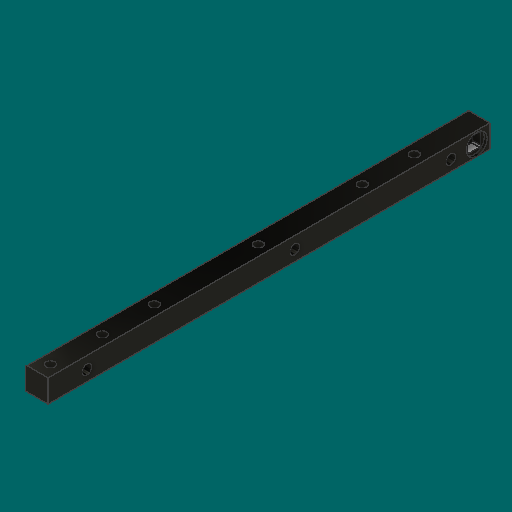
# Autodesk Inventor part: Intake_BOX
Saved by Autodesk Inventor 2025.2 (Build 292293000, 293)
## iProperties
Created: 2025-01-16
Part Number: Intake_BOX
Material: Generic
Document SubType Name: Modeling
Designer: Collin
Density: 1 g/cm^3
Appearance: Default
Author: Collin
Autodesk Inventor part; units mm, degrees
ref_plane "YZ Plane" through (0, 0, 0) normal (1, 0, 0) x (0, 1, 0)
ref_plane "XZ Plane" through (0, 0, 0) normal (0, 1, 0) x (-1, 0, 0)
ref_plane "XY Plane" through (0, 0, 0) normal (0, 0, 1) x (1, 0, 0)
sketch "Sketch1" plane through (0, 0, 0) normal (0, 1, 0) x (-1, 0, 0)
  point P0 (0, 0)
sketch "Sketch2" plane through (0, 0, 0) normal (0, 0, 1) x (1, 0, 0)
  line L0 (-7.0379, 7.3301) -> (-7.0379, 5.7426)
  line L1 (-7.0379, 7.3301) -> (-16.3407, 7.3301)
  line L2 (-16.3407, 7.3301) -> (-16.3407, 5.7426)
  line L3 (-16.3407, 5.7426) -> (-7.0379, 5.7426)
  arc A0 (-16.3407, 7.3301) -> (-18.7219, 4.9488) centre (-16.3407, 4.9488) ccw
  line L4 (-17.1344, 4.9488) -> (-18.7219, 4.9488)
  arc A1 (-16.3407, 5.7426) -> (-17.1344, 4.9488) centre (-16.3407, 4.9488) ccw
  line L5 (-16.3407, 7.3301) -> (-16.3407, 5.7426)
  arc A2 (-16.3407, 7.3301) -> (-18.7219, 4.9488) centre (-16.3407, 4.9488) ccw
  line L6 (-17.1344, 4.9488) -> (-18.7219, 4.9488)
  arc A3 (-16.3407, 5.7426) -> (-17.1344, 4.9488) centre (-16.3407, 4.9488) ccw
  line L7 (-7.0379, 7.3301) -> (-7.0379, 5.7426)
  line L8 (-7.0379, 7.3301) -> (-16.3407, 7.3301)
  line L9 (-16.3407, 5.7426) -> (-7.0379, 5.7426)
  line L10 (-18.7219, 2.1231) -> (-17.1344, 2.1231)
  line L11 (-17.1344, -4.3539) -> (-18.7219, -4.3539)
  line L12 (-17.1344, -4.3539) -> (-17.1344, 4.9488)
  line L13 (-17.1344, 4.9488) -> (-18.7219, 4.9488)
  line L14 (-18.7219, -4.3539) -> (-18.7219, 4.9488)
  line L15 (-17.1344, -5.3699) -> (-17.1344, -4.3539)
  line L16 (-17.1344, -4.3539) -> (-18.7219, -4.3539)
  line L17 (-18.7219, -4.3539) -> (-18.7219, -5.3699)
  line L18 (-18.7219, -5.3699) -> (-17.1344, -5.3699)
  line L19 (-6.0219, 7.3301) -> (-7.0379, 7.3301)
  line L20 (-7.0379, 7.3301) -> (-7.0379, 5.7426)
  line L21 (-7.0379, 5.7426) -> (-6.0219, 5.7426)
  line L22 (-6.0219, 5.7426) -> (-6.0219, 7.3301)
  line L23 (-17.1344, -5.3699) -> (-6.0219, -5.3699)
  line L24 (-6.0219, -5.3699) -> (-6.0219, 5.7426)
  point P0 (0, 0)
  point P1 (-18.7219, 0.9801)
  constraints: 50 end point, 8 point on circle, 4 centre point, 1 perpendicular
extrude "Extrusion1" add sketch "Sketch2" against normal blind 215.9 contours L21 L24 L23 L15 L12 A1 L3
sketch "Sketch3" plane through (-16.3407, 5.7426, 0) normal (0, 1, 0) x (1, 0, 0)
  line L0 (2.8257, 196.6074) -> (2.8257, 197.0926)
  line L1 (7.4485, 197.0926) -> (7.4485, 196.6074)
  line L2 (5.3798, 194.5386) -> (4.8945, 194.5386)
  line L3 (0, 215.9) -> (9.3027, 215.9)
  line L4 (0, 215.9) -> (0, 191.6657)
  line L5 (0, 191.6657) -> (1.1657, 190.5)
  line L6 (1.1657, 190.5) -> (0, 189.3343)
  line L7 (0, 189.3343) -> (0, 128.1657)
  line L8 (0, 128.1657) -> (1.1657, 127)
  line L9 (1.1657, 127) -> (0, 125.8343)
  line L10 (0, 125.8343) -> (0, 64.6657)
  line L11 (0, 64.6657) -> (1.1657, 63.5)
  line L12 (1.1657, 63.5) -> (0, 62.3343)
  line L13 (9.3027, 0) -> (0, 0)
  line L14 (10.3187, 61.468) -> (10.3187, 1.016)
  line L15 (10.3187, 61.468) -> (8.2867, 63.5)
  line L16 (8.2867, 63.5) -> (10.3187, 65.532)
  line L17 (10.3187, 124.968) -> (10.3187, 65.532)
  line L18 (10.3187, 124.968) -> (8.2867, 127)
  line L19 (8.2867, 127) -> (10.3187, 129.032)
  line L20 (10.3187, 188.468) -> (10.3187, 129.032)
  line L21 (10.3187, 188.468) -> (8.2867, 190.5)
  line L22 (8.2867, 190.5) -> (10.3187, 192.532)
  line L23 (10.3187, 214.884) -> (10.3187, 192.532)
  line L24 (-0.7938, 0) -> (0, 0)
  line L25 (0, 215.9) -> (10.3187, 215.9) projected
  line L26 (0, 215.9) -> (-0.7938, 215.9) projected
  line L27 (0, 0) -> (-0.7938, 0) projected
  line L28 (0, 0) -> (0, 215.9) projected
  line L29 (-0.7938, 215.9) -> (0, 215.9) projected
  line L30 (-0.7938, 0) -> (-0.7938, 215.9) projected
  line L31 (10.3187, 0) -> (0, 0) projected
  line L32 (10.3187, 0) -> (10.3187, 215.9) projected
  line L33 (0, 215.9) -> (10.3187, 215.9) projected
  line L34 (0, 0) -> (0, 215.9) projected
  line L35 (9.3027, 215.9) -> (10.3187, 215.9)
  line L36 (10.3187, 215.9) -> (10.3187, 214.884)
  line L37 (0, 62.3343) -> (0, 21.3614)
  line L38 (0, 16.7386) -> (0, 0)
  circle A0 centre (5.1371, 209.55) radius 2.161
  circle A1 centre (5.1371, 196.85) radius 2.161
  circle A2 centre (5.1371, 184.15) radius 2.161
  circle A3 centre (5.1371, 171.45) radius 2.161
  circle A4 centre (5.1371, 158.75) radius 2.161
  circle A5 centre (5.1371, 146.05) radius 2.161
  circle A6 centre (5.1371, 133.35) radius 2.161
  circle A7 centre (5.1371, 120.65) radius 2.161
  circle A8 centre (5.1371, 107.95) radius 2.161
  circle A9 centre (5.1371, 95.25) radius 2.161
  circle A10 centre (5.1371, 82.55) radius 2.161
  circle A11 centre (5.1371, 69.85) radius 2.161
  circle A12 centre (5.1371, 57.15) radius 2.161
  circle A13 centre (5.1371, 44.45) radius 2.161
  circle A14 centre (5.1371, 31.75) radius 2.161
  circle A15 centre (5.1371, 19.05) radius 2.161
  circle A16 centre (5.1371, 6.35) radius 2.161
  point P0 (16.3407, 0)
  dimension "d9" = 12.7
  constraints: 58 end point, 17 centre point, 1 horizontal, 1 perpendicular, 1 point on line, 1 vertical, 32 other
  measures "d9" distance of A0.centre A1.centre
extrude "Extrusion2" cut sketch "Sketch3" along normal mid plane 215.9 contours A2 | A4 | A8 | A12 | A14 | A16
sketch "Sketch4" plane through (-6.0219, -5.3699, 0) normal (1, 0, 0) x (0, 0, -1)
  line L0 (0, 0) -> (0, 11.1125)
  line L1 (0, 0) -> (215.9, 0)
  line L2 (215.9, 11.1125) -> (215.9, 0)
  line L3 (0, 11.1125) -> (215.9, 11.1125)
  arc A0 (4.5466, 7.493) -> (4.0386, 6.985) centre (4.5466, 6.985) ccw
  line L4 (4.5466, 7.493) -> (8.1534, 7.493)
  arc A1 (8.6614, 6.985) -> (8.1534, 7.493) centre (8.1534, 6.985) ccw
  line L5 (8.6614, 6.985) -> (8.6614, 3.3782)
  arc A2 (8.1534, 2.8702) -> (8.6614, 3.3782) centre (8.1534, 3.3782) ccw
  line L6 (8.1534, 2.8702) -> (4.5466, 2.8702)
  arc A3 (4.0386, 3.3782) -> (4.5466, 2.8702) centre (4.5466, 3.3782) ccw
  line L7 (4.0386, 3.3782) -> (4.0386, 6.985)
  arc A4 (29.9466, 7.493) -> (29.4386, 6.985) centre (29.9466, 6.985) ccw
  line L8 (29.9466, 7.493) -> (33.5534, 7.493)
  arc A5 (34.0614, 6.985) -> (33.5534, 7.493) centre (33.5534, 6.985) ccw
  line L9 (34.0614, 6.985) -> (34.0614, 3.3782)
  arc A6 (33.5534, 2.8702) -> (34.0614, 3.3782) centre (33.5534, 3.3782) ccw
  line L10 (33.5534, 2.8702) -> (29.9466, 2.8702)
  arc A7 (29.4386, 3.3782) -> (29.9466, 2.8702) centre (29.9466, 3.3782) ccw
  line L11 (29.4386, 3.3782) -> (29.4386, 6.985)
  arc A8 (42.6466, 7.493) -> (42.1386, 6.985) centre (42.6466, 6.985) ccw
  line L12 (42.6466, 7.493) -> (46.2534, 7.493)
  arc A9 (46.7614, 6.985) -> (46.2534, 7.493) centre (46.2534, 6.985) ccw
  line L13 (46.7614, 6.985) -> (46.7614, 3.3782)
  arc A10 (46.2534, 2.8702) -> (46.7614, 3.3782) centre (46.2534, 3.3782) ccw
  line L14 (46.2534, 2.8702) -> (42.6466, 2.8702)
  arc A11 (42.1386, 3.3782) -> (42.6466, 2.8702) centre (42.6466, 3.3782) ccw
  line L15 (42.1386, 3.3782) -> (42.1386, 6.985)
  arc A12 (55.3466, 7.493) -> (54.8386, 6.985) centre (55.3466, 6.985) ccw
  line L16 (55.3466, 7.493) -> (58.9534, 7.493)
  arc A13 (59.4614, 6.985) -> (58.9534, 7.493) centre (58.9534, 6.985) ccw
  line L17 (59.4614, 6.985) -> (59.4614, 3.3782)
  arc A14 (58.9534, 2.8702) -> (59.4614, 3.3782) centre (58.9534, 3.3782) ccw
  line L18 (58.9534, 2.8702) -> (55.3466, 2.8702)
  arc A15 (54.8386, 3.3782) -> (55.3466, 2.8702) centre (55.3466, 3.3782) ccw
  line L19 (54.8386, 3.3782) -> (54.8386, 6.985)
  arc A16 (68.0466, 7.493) -> (67.5386, 6.985) centre (68.0466, 6.985) ccw
  line L20 (68.0466, 7.493) -> (71.6534, 7.493)
  arc A17 (72.1614, 6.985) -> (71.6534, 7.493) centre (71.6534, 6.985) ccw
  line L21 (72.1614, 6.985) -> (72.1614, 3.3782)
  arc A18 (71.6534, 2.8702) -> (72.1614, 3.3782) centre (71.6534, 3.3782) ccw
  line L22 (71.6534, 2.8702) -> (68.0466, 2.8702)
  arc A19 (67.5386, 3.3782) -> (68.0466, 2.8702) centre (68.0466, 3.3782) ccw
  line L23 (67.5386, 3.3782) -> (67.5386, 6.985)
  arc A20 (80.7466, 7.493) -> (80.2386, 6.985) centre (80.7466, 6.985) ccw
  line L24 (80.7466, 7.493) -> (84.3534, 7.493)
  arc A21 (84.8614, 6.985) -> (84.3534, 7.493) centre (84.3534, 6.985) ccw
  line L25 (84.8614, 6.985) -> (84.8614, 3.3782)
  arc A22 (84.3534, 2.8702) -> (84.8614, 3.3782) centre (84.3534, 3.3782) ccw
  line L26 (84.3534, 2.8702) -> (80.7466, 2.8702)
  arc A23 (80.2386, 3.3782) -> (80.7466, 2.8702) centre (80.7466, 3.3782) ccw
  line L27 (80.2386, 3.3782) -> (80.2386, 6.985)
  arc A24 (93.4466, 7.493) -> (92.9386, 6.985) centre (93.4466, 6.985) ccw
  line L28 (93.4466, 7.493) -> (97.0534, 7.493)
  arc A25 (97.5614, 6.985) -> (97.0534, 7.493) centre (97.0534, 6.985) ccw
  line L29 (97.5614, 6.985) -> (97.5614, 3.3782)
  arc A26 (97.0534, 2.8702) -> (97.5614, 3.3782) centre (97.0534, 3.3782) ccw
  line L30 (97.0534, 2.8702) -> (93.4466, 2.8702)
  arc A27 (92.9386, 3.3782) -> (93.4466, 2.8702) centre (93.4466, 3.3782) ccw
  line L31 (92.9386, 3.3782) -> (92.9386, 6.985)
  arc A28 (106.1466, 7.493) -> (105.6386, 6.985) centre (106.1466, 6.985) ccw
  line L32 (106.1466, 7.493) -> (109.7534, 7.493)
  arc A29 (110.2614, 6.985) -> (109.7534, 7.493) centre (109.7534, 6.985) ccw
  line L33 (110.2614, 6.985) -> (110.2614, 3.3782)
  arc A30 (109.7534, 2.8702) -> (110.2614, 3.3782) centre (109.7534, 3.3782) ccw
  line L34 (109.7534, 2.8702) -> (106.1466, 2.8702)
  arc A31 (105.6386, 3.3782) -> (106.1466, 2.8702) centre (106.1466, 3.3782) ccw
  line L35 (105.6386, 3.3782) -> (105.6386, 6.985)
  line L36 (120.4074, 7.493) -> (120.8926, 7.493)
  arc A32 (131.5466, 7.493) -> (131.0386, 6.985) centre (131.5466, 6.985) ccw
  line L37 (131.5466, 7.493) -> (135.1534, 7.493)
  arc A33 (135.6614, 6.985) -> (135.1534, 7.493) centre (135.1534, 6.985) ccw
  line L38 (135.6614, 6.985) -> (135.6614, 3.3782)
  arc A34 (135.1534, 2.8702) -> (135.6614, 3.3782) centre (135.1534, 3.3782) ccw
  line L39 (135.1534, 2.8702) -> (131.5466, 2.8702)
  arc A35 (131.0386, 3.3782) -> (131.5466, 2.8702) centre (131.5466, 3.3782) ccw
  line L40 (131.0386, 3.3782) -> (131.0386, 6.985)
  arc A36 (144.2466, 7.493) -> (143.7386, 6.985) centre (144.2466, 6.985) ccw
  line L41 (144.2466, 7.493) -> (147.8534, 7.493)
  arc A37 (148.3614, 6.985) -> (147.8534, 7.493) centre (147.8534, 6.985) ccw
  line L42 (148.3614, 6.985) -> (148.3614, 3.3782)
  arc A38 (147.8534, 2.8702) -> (148.3614, 3.3782) centre (147.8534, 3.3782) ccw
  line L43 (147.8534, 2.8702) -> (144.2466, 2.8702)
  arc A39 (143.7386, 3.3782) -> (144.2466, 2.8702) centre (144.2466, 3.3782) ccw
  line L44 (143.7386, 3.3782) -> (143.7386, 6.985)
  arc A40 (156.9466, 7.493) -> (156.4386, 6.985) centre (156.9466, 6.985) ccw
  line L45 (156.9466, 7.493) -> (160.5534, 7.493)
  arc A41 (161.0614, 6.985) -> (160.5534, 7.493) centre (160.5534, 6.985) ccw
  line L46 (161.0614, 6.985) -> (161.0614, 3.3782)
  arc A42 (160.5534, 2.8702) -> (161.0614, 3.3782) centre (160.5534, 3.3782) ccw
  line L47 (160.5534, 2.8702) -> (156.9466, 2.8702)
  arc A43 (156.4386, 3.3782) -> (156.9466, 2.8702) centre (156.9466, 3.3782) ccw
  line L48 (156.4386, 3.3782) -> (156.4386, 6.985)
  arc A44 (169.6466, 7.493) -> (169.1386, 6.985) centre (169.6466, 6.985) ccw
  line L49 (169.6466, 7.493) -> (173.2534, 7.493)
  arc A45 (173.7614, 6.985) -> (173.2534, 7.493) centre (173.2534, 6.985) ccw
  line L50 (173.7614, 6.985) -> (173.7614, 3.3782)
  arc A46 (173.2534, 2.8702) -> (173.7614, 3.3782) centre (173.2534, 3.3782) ccw
  line L51 (173.2534, 2.8702) -> (169.6466, 2.8702)
  arc A47 (169.1386, 3.3782) -> (169.6466, 2.8702) centre (169.6466, 3.3782) ccw
  line L52 (169.1386, 3.3782) -> (169.1386, 6.985)
  arc A48 (182.3466, 7.493) -> (181.8386, 6.985) centre (182.3466, 6.985) ccw
  line L53 (182.3466, 7.493) -> (185.9534, 7.493)
  arc A49 (186.4614, 6.985) -> (185.9534, 7.493) centre (185.9534, 6.985) ccw
  line L54 (186.4614, 6.985) -> (186.4614, 3.3782)
  arc A50 (185.9534, 2.8702) -> (186.4614, 3.3782) centre (185.9534, 3.3782) ccw
  line L55 (185.9534, 2.8702) -> (182.3466, 2.8702)
  arc A51 (181.8386, 3.3782) -> (182.3466, 2.8702) centre (182.3466, 3.3782) ccw
  line L56 (181.8386, 3.3782) -> (181.8386, 6.985)
  arc A52 (207.7466, 7.493) -> (207.2386, 6.985) centre (207.7466, 6.985) ccw
  line L57 (207.7466, 7.493) -> (211.3534, 7.493)
  arc A53 (211.8614, 6.985) -> (211.3534, 7.493) centre (211.3534, 6.985) ccw
  line L58 (211.8614, 6.985) -> (211.8614, 3.3782)
  arc A54 (211.3534, 2.8702) -> (211.8614, 3.3782) centre (211.3534, 3.3782) ccw
  line L59 (211.3534, 2.8702) -> (207.7466, 2.8702)
  arc A55 (207.2386, 3.3782) -> (207.7466, 2.8702) centre (207.7466, 3.3782) ccw
  line L60 (207.2386, 3.3782) -> (207.2386, 6.985)
  line L61 (215.9, 10.3187) -> (215.9, 1.016)
  line L62 (215.9, 10.3187) -> (191.6657, 10.3187)
  line L63 (189.3343, 10.3187) -> (128.1657, 10.3187)
  line L64 (125.8343, 10.3187) -> (64.6657, 10.3187)
  line L65 (62.3343, 10.3187) -> (0, 10.3187)
  line L66 (0, 1.016) -> (0, 10.3187)
  line L67 (61.468, 0) -> (1.016, 0)
  line L68 (124.968, 0) -> (65.532, 0)
  line L69 (188.468, 0) -> (129.032, 0)
  line L70 (214.884, 0) -> (192.532, 0)
  line L71 (1.016, 12.7) -> (0, 12.7)
  line L72 (0, 12.7) -> (0, 11.1125)
  line L73 (0, 11.1125) -> (1.016, 11.1125)
  line L74 (1.016, 11.1125) -> (1.016, 12.7)
  spline S0 degree 3 poles (61.2372, 10.9075) (61.6029, 11.0379) (61.9686, 11.1125) (62.3343, 11.1125) knots -1 -1 -1 -1 0 0 0 0
  line L75 (0, 11.1125) -> (62.3343, 11.1125)
  line L76 (0, 10.3187) -> (0, 11.1125)
  line L77 (62.3343, 10.3187) -> (0, 10.3187)
  spline S1 degree 3 poles (62.3343, 10.3187) (61.9686, 10.5133) (61.6029, 10.7069) (61.2372, 10.8512) knots 0 0 0 0 1 1 1 1
  spline S2 degree 3 poles (61.2372, 10.8512) (61.2621, 10.861) (61.2871, 10.8706) (61.312, 10.88) knots 0 0 0 0 1 1 1 1
  spline S3 degree 3 poles (61.312, 10.88) (61.2871, 10.8894) (61.2621, 10.8985) (61.2372, 10.9075) knots 0 0 0 0 1 1 1 1
  line L78 (1.016, 11.1125) -> (1.016, 12.7)
  line L79 (61.468, 11.1125) -> (1.016, 11.1125)
  line L80 (61.468, 11.1125) -> (61.468, 12.7)
  line L81 (61.468, 12.7) -> (1.016, 12.7)
  line L82 (63.5, 11.1125) -> (61.468, 11.1125)
  line L83 (63.5, 12.7) -> (63.5, 11.1125)
  line L84 (61.468, 12.7) -> (63.5, 12.7)
  line L85 (61.468, 11.1125) -> (61.468, 12.7)
  line L86 (65.532, 11.1125) -> (63.5, 11.1125)
  line L87 (65.532, 12.7) -> (65.532, 11.1125)
  line L88 (63.5, 12.7) -> (65.532, 12.7)
  line L89 (63.5, 12.7) -> (63.5, 11.1125)
  line L90 (68.0466, 12.7) -> (68.0466, 11.1125)
  line L91 (124.968, 11.1125) -> (124.968, 12.7)
  line L92 (124.968, 12.7) -> (65.532, 12.7)
  line L93 (65.532, 12.7) -> (65.532, 11.1125)
  line L94 (124.968, 11.1125) -> (65.532, 11.1125)
  spline S4 degree 3 poles (124.7372, 10.9075) (125.1029, 11.0379) (125.4686, 11.1125) (125.8343, 11.1125) knots -1 -1 -1 -1 0 0 0 0
  line L95 (64.6657, 11.1125) -> (125.8343, 11.1125)
  spline S5 degree 3 poles (64.6657, 11.1125) (65.0314, 11.1125) (65.3971, 11.0379) (65.7628, 10.9075) knots -1 -1 -1 -1 0 0 0 0
  spline S6 degree 3 poles (65.7628, 10.9075) (65.7379, 10.8985) (65.7129, 10.8894) (65.688, 10.88) knots 0 0 0 0 1 1 1 1
  spline S7 degree 3 poles (65.688, 10.88) (65.7129, 10.8706) (65.7379, 10.861) (65.7628, 10.8512) knots 0 0 0 0 1 1 1 1
  spline S8 degree 3 poles (65.7628, 10.8512) (65.3971, 10.7069) (65.0314, 10.5133) (64.6657, 10.3187) knots 0 0 0 0 1 1 1 1
  line L96 (125.8343, 10.3187) -> (64.6657, 10.3187)
  spline S9 degree 3 poles (125.8343, 10.3187) (125.4686, 10.5133) (125.1029, 10.7069) (124.7372, 10.8512) knots 0 0 0 0 1 1 1 1
  spline S10 degree 3 poles (124.7372, 10.8512) (124.7621, 10.861) (124.7871, 10.8706) (124.812, 10.88) knots 0 0 0 0 1 1 1 1
  spline S11 degree 3 poles (124.812, 10.88) (124.7871, 10.8894) (124.7621, 10.8985) (124.7372, 10.9075) knots 0 0 0 0 1 1 1 1
  line L97 (129.032, 11.1125) -> (127, 11.1125)
  line L98 (129.032, 12.7) -> (129.032, 11.1125)
  line L99 (127, 12.7) -> (129.032, 12.7)
  line L100 (127, 12.7) -> (127, 11.1125)
  line L101 (127, 11.1125) -> (124.968, 11.1125)
  line L102 (127, 12.7) -> (127, 11.1125)
  line L103 (124.968, 12.7) -> (127, 12.7)
  line L104 (124.968, 11.1125) -> (124.968, 12.7)
  line L105 (129.032, 12.7) -> (129.032, 11.1125)
  line L106 (188.468, 11.1125) -> (129.032, 11.1125)
  line L107 (188.468, 11.1125) -> (188.468, 12.7)
  line L108 (188.468, 12.7) -> (129.032, 12.7)
  spline S12 degree 3 poles (128.1657, 11.1125) (128.5314, 11.1125) (128.8971, 11.0379) (129.2628, 10.9075) knots -1 -1 -1 -1 0 0 0 0
  spline S13 degree 3 poles (129.2628, 10.9075) (129.2379, 10.8985) (129.2129, 10.8894) (129.188, 10.88) knots 0 0 0 0 1 1 1 1
  spline S14 degree 3 poles (129.188, 10.88) (129.2129, 10.8706) (129.2379, 10.861) (129.2628, 10.8512) knots 0 0 0 0 1 1 1 1
  spline S15 degree 3 poles (129.2628, 10.8512) (128.8971, 10.7069) (128.5314, 10.5133) (128.1657, 10.3187) knots 0 0 0 0 1 1 1 1
  line L109 (189.3343, 10.3187) -> (128.1657, 10.3187)
  spline S16 degree 3 poles (189.3343, 10.3187) (188.9686, 10.5133) (188.6029, 10.7069) (188.2372, 10.8512) knots 0 0 0 0 1 1 1 1
  spline S17 degree 3 poles (188.2372, 10.8512) (188.2621, 10.861) (188.2871, 10.8706) (188.312, 10.88) knots 0 0 0 0 1 1 1 1
  spline S18 degree 3 poles (188.312, 10.88) (188.2871, 10.8894) (188.2621, 10.8985) (188.2372, 10.9075) knots 0 0 0 0 1 1 1 1
  spline S19 degree 3 poles (188.2372, 10.9075) (188.6029, 11.0379) (188.9686, 11.1125) (189.3343, 11.1125) knots -1 -1 -1 -1 0 0 0 0
  line L110 (128.1657, 11.1125) -> (189.3343, 11.1125)
  line L111 (190.5, 11.1125) -> (188.468, 11.1125)
  line L112 (190.5, 12.7) -> (190.5, 11.1125)
  line L113 (188.468, 12.7) -> (190.5, 12.7)
  line L114 (188.468, 11.1125) -> (188.468, 12.7)
  line L115 (192.532, 11.1125) -> (190.5, 11.1125)
  line L116 (192.532, 12.7) -> (192.532, 11.1125)
  line L117 (190.5, 12.7) -> (192.532, 12.7)
  line L118 (190.5, 12.7) -> (190.5, 11.1125)
  line L119 (214.884, 12.7) -> (214.884, 11.1125)
  line L120 (214.884, 12.7) -> (192.532, 12.7)
  line L121 (192.532, 12.7) -> (192.532, 11.1125)
  line L122 (214.884, 11.1125) -> (192.532, 11.1125)
  spline S20 degree 3 poles (192.7628, 10.9075) (192.7379, 10.8985) (192.7129, 10.8894) (192.688, 10.88) knots 0 0 0 0 1 1 1 1
  spline S21 degree 3 poles (192.688, 10.88) (192.7129, 10.8706) (192.7379, 10.861) (192.7628, 10.8512) knots 0 0 0 0 1 1 1 1
  spline S22 degree 3 poles (192.7628, 10.8512) (192.3971, 10.7069) (192.0314, 10.5133) (191.6657, 10.3187) knots 0 0 0 0 1 1 1 1
  line L123 (215.9, 10.3187) -> (191.6657, 10.3187)
  line L124 (215.9, 10.3187) -> (215.9, 11.1125)
  line L125 (191.6657, 11.1125) -> (215.9, 11.1125)
  spline S23 degree 3 poles (191.6657, 11.1125) (192.0314, 11.1125) (192.3971, 11.0379) (192.7628, 10.9075) knots -1 -1 -1 -1 0 0 0 0
  line L126 (215.9, 12.7) -> (214.884, 12.7)
  line L127 (214.884, 12.7) -> (214.884, 11.1125)
  line L128 (214.884, 11.1125) -> (215.9, 11.1125)
  line L129 (215.9, 11.1125) -> (215.9, 12.7)
  circle A56 centre (120.65, 5.1816) radius 2.3241
  circle A57 centre (196.85, 5.1816) radius 2.3241
  circle A58 centre (19.05, 5.1816) radius 2.3241
  point P0 (0, 5.3699)
  point P1 (0, 6.35)
  point P2 (125.8343, 11.811)
  dimension "d16" = 4.6482
  dimension "d17" = 4.6482
  dimension "d18" = 4.6482
  constraints: 252 end point, 114 point on circle, 59 centre point, 72 other
  measures "d16" diameter of A56
  measures "d17" diameter of A57
  measures "d18" diameter of A58
extrude "Extrusion3" cut sketch "Sketch4" along normal through all both and the other way through all contours L36 A56 | A57 | A58 picked at (121.7622, 5.7025)
sketch "Sketch5" plane through (-17.1344, -5.3699, 0) normal (-1, 0, 0) x (0, 0, 1)
  circle A0 centre (-196.85, 5.1816) radius 2.3241 projected
  arc A1 (-120.8926, 7.493) -> (-120.4074, 7.493) centre (-120.65, 5.1816) ccw projected
  line L0 (-120.8926, 7.493) -> (-120.4074, 7.493) projected
  circle A2 centre (-19.05, 5.1816) radius 2.3241 projected
  line L1 (0, 10.3187) -> (0, 0) projected
  line L2 (0, 10.3187) -> (-215.9, 10.3187) projected
  line L3 (-215.9, 0) -> (-215.9, 10.3187) projected
  line L4 (0, 0) -> (-215.9, 0) projected
  line L5 (-214.884, 0) -> (-215.9, 1.016)
  line L6 (-214.884, 0) -> (-192.532, 0)
  line L7 (-192.532, 0) -> (-190.5, 2.032)
  line L8 (-190.5, 2.032) -> (-188.468, 0)
  line L9 (-188.468, 0) -> (-129.032, 0)
  line L10 (-129.032, 0) -> (-127, 2.032)
  line L11 (-127, 2.032) -> (-124.968, 0)
  line L12 (-124.968, 0) -> (-65.532, 0)
  line L13 (-65.532, 0) -> (-63.5, 2.032)
  line L14 (-63.5, 2.032) -> (-61.468, 0)
  line L15 (-61.468, 0) -> (-1.016, 0)
  line L16 (0, 1.016) -> (0, 10.3187)
  line L17 (0, 10.3187) -> (-62.3343, 10.3187)
  line L18 (-62.3343, 10.3187) -> (-63.5, 9.1531)
  line L19 (-63.5, 9.1531) -> (-64.6657, 10.3187)
  line L20 (-64.6657, 10.3187) -> (-125.8343, 10.3187)
  line L21 (-125.8343, 10.3187) -> (-127, 9.1531)
  line L22 (-127, 9.1531) -> (-128.1657, 10.3187)
  line L23 (-128.1657, 10.3187) -> (-189.3343, 10.3187)
  line L24 (-189.3343, 10.3187) -> (-190.5, 9.1531)
  line L25 (-190.5, 9.1531) -> (-191.6657, 10.3188)
  line L26 (-191.6657, 10.3188) -> (-215.9, 10.3187)
  line L27 (-215.9, 10.3187) -> (-215.9, 1.016)
  arc A3 (-16.7386, 6.985) -> (-17.2466, 7.493) centre (-17.2466, 6.985) ccw
  line L28 (-16.7386, 6.985) -> (-16.7386, 3.3782)
  arc A4 (-17.2466, 2.8702) -> (-16.7386, 3.3782) centre (-17.2466, 3.3782) ccw
  line L29 (-17.2466, 2.8702) -> (-20.8534, 2.8702)
  arc A5 (-21.3614, 3.3782) -> (-20.8534, 2.8702) centre (-20.8534, 3.3782) ccw
  line L30 (-21.3614, 3.3782) -> (-21.3614, 6.985)
  arc A6 (-20.8534, 7.493) -> (-21.3614, 6.985) centre (-20.8534, 6.985) ccw
  line L31 (-20.8534, 7.493) -> (-17.2466, 7.493)
  arc A7 (-118.3386, 6.985) -> (-118.8466, 7.493) centre (-118.8466, 6.985) ccw
  line L32 (-118.3386, 6.985) -> (-118.3386, 3.3782)
  arc A8 (-118.8466, 2.8702) -> (-118.3386, 3.3782) centre (-118.8466, 3.3782) ccw
  line L33 (-118.8466, 2.8702) -> (-122.4534, 2.8702)
  arc A9 (-122.9614, 3.3782) -> (-122.4534, 2.8702) centre (-122.4534, 3.3782) ccw
  line L34 (-122.9614, 3.3782) -> (-122.9614, 6.985)
  arc A10 (-122.4534, 7.493) -> (-122.9614, 6.985) centre (-122.4534, 6.985) ccw
  line L35 (-122.4534, 7.493) -> (-118.8466, 7.493)
  line L36 (-191.6657, 11.1125) -> (-215.9, 11.1125)
  line L37 (-128.1657, 11.1125) -> (-189.3343, 11.1125)
  line L38 (-64.6657, 11.1125) -> (-125.8343, 11.1125)
  line L39 (0, 11.1125) -> (-62.3343, 11.1125)
  line L40 (-1.016, 0) -> (0, 0)
  line L41 (0, 0) -> (0, 1.016)
  line L42 (-7.3025, 7.4041) -> (-5.3975, 7.4041)
  line L43 (-4.1275, 6.1341) -> (-4.1275, 4.2291)
  line L44 (-5.3975, 2.9591) -> (-7.3025, 2.9591)
  line L45 (-8.5725, 4.2291) -> (-8.5725, 6.1341)
  arc A11 (-7.3025, 7.4041) -> (-8.5725, 6.1341) centre (-7.3025, 6.1341) ccw
  arc A12 (-4.1275, 6.1341) -> (-5.3975, 7.4041) centre (-5.3975, 6.1341) ccw
  arc A13 (-5.3975, 2.9591) -> (-4.1275, 4.2291) centre (-5.3975, 4.2291) ccw
  arc A14 (-8.5725, 4.2291) -> (-7.3025, 2.9591) centre (-7.3025, 4.2291) ccw
  arc A15 (-32.7025, 7.4041) -> (-33.9725, 6.1341) centre (-32.7025, 6.1341) ccw
  line L46 (-32.7025, 7.4041) -> (-30.7975, 7.4041)
  arc A16 (-29.5275, 6.1341) -> (-30.7975, 7.4041) centre (-30.7975, 6.1341) ccw
  line L47 (-29.5275, 6.1341) -> (-29.5275, 4.2291)
  arc A17 (-30.7975, 2.9591) -> (-29.5275, 4.2291) centre (-30.7975, 4.2291) ccw
  line L48 (-30.7975, 2.9591) -> (-32.7025, 2.9591)
  arc A18 (-33.9725, 4.2291) -> (-32.7025, 2.9591) centre (-32.7025, 4.2291) ccw
  line L49 (-33.9725, 4.2291) -> (-33.9725, 6.1341)
  arc A19 (-58.1025, 7.4041) -> (-59.3725, 6.1341) centre (-58.1025, 6.1341) ccw
  line L50 (-58.1025, 7.4041) -> (-56.1975, 7.4041)
  arc A20 (-54.9275, 6.1341) -> (-56.1975, 7.4041) centre (-56.1975, 6.1341) ccw
  line L51 (-54.9275, 6.1341) -> (-54.9275, 4.2291)
  arc A21 (-56.1975, 2.9591) -> (-54.9275, 4.2291) centre (-56.1975, 4.2291) ccw
  line L52 (-56.1975, 2.9591) -> (-58.1025, 2.9591)
  arc A22 (-59.3725, 4.2291) -> (-58.1025, 2.9591) centre (-58.1025, 4.2291) ccw
  line L53 (-59.3725, 4.2291) -> (-59.3725, 6.1341)
  arc A23 (-83.5025, 7.4041) -> (-84.7725, 6.1341) centre (-83.5025, 6.1341) ccw
  line L54 (-83.5025, 7.4041) -> (-81.5975, 7.4041)
  arc A24 (-80.3275, 6.1341) -> (-81.5975, 7.4041) centre (-81.5975, 6.1341) ccw
  line L55 (-80.3275, 6.1341) -> (-80.3275, 4.2291)
  arc A25 (-81.5975, 2.9591) -> (-80.3275, 4.2291) centre (-81.5975, 4.2291) ccw
  line L56 (-81.5975, 2.9591) -> (-83.5025, 2.9591)
  arc A26 (-84.7725, 4.2291) -> (-83.5025, 2.9591) centre (-83.5025, 4.2291) ccw
  line L57 (-84.7725, 4.2291) -> (-84.7725, 6.1341)
  arc A27 (-108.9025, 7.4041) -> (-110.1725, 6.1341) centre (-108.9025, 6.1341) ccw
  line L58 (-108.9025, 7.4041) -> (-106.9975, 7.4041)
  arc A28 (-105.7275, 6.1341) -> (-106.9975, 7.4041) centre (-106.9975, 6.1341) ccw
  line L59 (-105.7275, 6.1341) -> (-105.7275, 4.2291)
  arc A29 (-106.9975, 2.9591) -> (-105.7275, 4.2291) centre (-106.9975, 4.2291) ccw
  line L60 (-106.9975, 2.9591) -> (-108.9025, 2.9591)
  arc A30 (-110.1725, 4.2291) -> (-108.9025, 2.9591) centre (-108.9025, 4.2291) ccw
  line L61 (-110.1725, 4.2291) -> (-110.1725, 6.1341)
  arc A31 (-134.3025, 7.4041) -> (-135.5725, 6.1341) centre (-134.3025, 6.1341) ccw
  line L62 (-134.3025, 7.4041) -> (-132.3975, 7.4041)
  arc A32 (-131.1275, 6.1341) -> (-132.3975, 7.4041) centre (-132.3975, 6.1341) ccw
  line L63 (-131.1275, 6.1341) -> (-131.1275, 4.2291)
  arc A33 (-132.3975, 2.9591) -> (-131.1275, 4.2291) centre (-132.3975, 4.2291) ccw
  line L64 (-132.3975, 2.9591) -> (-134.3025, 2.9591)
  arc A34 (-135.5725, 4.2291) -> (-134.3025, 2.9591) centre (-134.3025, 4.2291) ccw
  line L65 (-135.5725, 4.2291) -> (-135.5725, 6.1341)
  arc A35 (-159.7025, 7.4041) -> (-160.9725, 6.1341) centre (-159.7025, 6.1341) ccw
  line L66 (-159.7025, 7.4041) -> (-157.7975, 7.4041)
  arc A36 (-156.5275, 6.1341) -> (-157.7975, 7.4041) centre (-157.7975, 6.1341) ccw
  line L67 (-156.5275, 6.1341) -> (-156.5275, 4.2291)
  arc A37 (-157.7975, 2.9591) -> (-156.5275, 4.2291) centre (-157.7975, 4.2291) ccw
  line L68 (-157.7975, 2.9591) -> (-159.7025, 2.9591)
  arc A38 (-160.9725, 4.2291) -> (-159.7025, 2.9591) centre (-159.7025, 4.2291) ccw
  line L69 (-160.9725, 4.2291) -> (-160.9725, 6.1341)
  arc A39 (-185.1025, 7.4041) -> (-186.3725, 6.1341) centre (-185.1025, 6.1341) ccw
  line L70 (-185.1025, 7.4041) -> (-183.1975, 7.4041)
  arc A40 (-181.9275, 6.1341) -> (-183.1975, 7.4041) centre (-183.1975, 6.1341) ccw
  line L71 (-181.9275, 6.1341) -> (-181.9275, 4.2291)
  arc A41 (-183.1975, 2.9591) -> (-181.9275, 4.2291) centre (-183.1975, 4.2291) ccw
  line L72 (-183.1975, 2.9591) -> (-185.1025, 2.9591)
  arc A42 (-186.3725, 4.2291) -> (-185.1025, 2.9591) centre (-185.1025, 4.2291) ccw
  line L73 (-186.3725, 4.2291) -> (-186.3725, 6.1341)
  arc A43 (-210.5025, 7.4041) -> (-211.7725, 6.1341) centre (-210.5025, 6.1341) ccw
  line L74 (-210.5025, 7.4041) -> (-208.5975, 7.4041)
  arc A44 (-207.3275, 6.1341) -> (-208.5975, 7.4041) centre (-208.5975, 6.1341) ccw
  line L75 (-207.3275, 6.1341) -> (-207.3275, 4.2291)
  arc A45 (-208.5975, 2.9591) -> (-207.3275, 4.2291) centre (-208.5975, 4.2291) ccw
  line L76 (-208.5975, 2.9591) -> (-210.5025, 2.9591)
  arc A46 (-211.7725, 4.2291) -> (-210.5025, 2.9591) centre (-210.5025, 4.2291) ccw
  line L77 (-211.7725, 4.2291) -> (-211.7725, 6.1341)
  point P0 (0, 5.3699)
  point P1 (0, 6.35)
  dimension "d22" = 1.27
  dimension "d25" = 25.4
  constraints: 146 end point, 88 point on circle, 44 centre point, 8 tangent, 3 equal radius, 3 horizontal, 2 parallel, 2 perpendicular, 160 other
  measures "d22" radius of A11
  measures "d25" distance of A11.centre A15.centre
extrude "Extrusion4" add sketch "Sketch5" along normal blind 1.5875 contours L42 A12 L43 A13 L44 A14 L45 A11 | L46 A16 L47 A17 L48 A18 L49 A15 | L50 A20 L51 A21 L52 A22 L53 A19 | L54 A24 L55 A25 L56 A26 L57 A23 | L58 A28 L59 A29 L60 A30 L61 A27 | L62 A32 L63 A33 L64 A34 L65 A31 | L66 A36 L67 A37 L68 A38 L69 A35 | L70 A40 L71 A41 L72 A42 L73 A39 | L74 A44 L75 A45 L76 A46 L77 A43
sketch "Sketch6" plane through (-6.0219, -5.3699, 0) normal (1, 0, 0) x (0, 0, -1)
  circle A0 centre (196.85, 5.1816) radius 2.3241 projected
  arc A1 (120.4074, 7.493) -> (120.8926, 7.493) centre (120.65, 5.1816) ccw projected
  line L0 (120.4074, 7.493) -> (120.8926, 7.493) projected
  circle A2 centre (19.05, 5.1816) radius 2.3241 projected
  line L1 (0, 0) -> (0, 11.1125) projected
  line L2 (0, 0) -> (215.9, 0) projected
  line L3 (215.9, 11.1125) -> (215.9, 0) projected
  line L4 (0, 11.1125) -> (215.9, 11.1125) projected
  line L5 (196.85, 5.1816) -> (209.55, 5.1816)
  circle A3 centre (209.55, 5.1816) radius 5.08
  line L6 (209.55, 5.1816) -> (209.55, 10.2616)
  line L7 (209.55, 5.1816) -> (209.55, 0.1016)
  line L8 (209.55, 0.1016) -> (209.55, -0.254)
  point P0 (0, 5.3699)
  dimension "d32" = 12.7
  dimension "d33" = 10.16
  dimension "d36" = 0.3556
  constraints: 8 end point, 2 point on circle, 2 vertical, 1 centre point, 1 coincident, 1 horizontal, 1 perpendicular
  measures "d32" distance of L5.start L5.end
  measures "d33" diameter of A3
  measures "d36" distance of L7.end L8.end
extrude "Extrusion5" cut sketch "Sketch6" against normal blind 1.397 contours A3 L6 L5 | L5 L7 A3 | L6 A3 L7
sketch "Sketch7" plane through (-17.1344, -5.3699, 0) normal (0, -1, 0) x (1, 0, 0)
  circle A0 centre (5.9309, -57.15) radius 2.161 projected
  circle A1 centre (5.9309, -184.15) radius 2.161 projected
  circle A2 centre (5.9309, -31.75) radius 2.161 projected
  circle A3 centre (5.9309, -107.95) radius 2.161 projected
  circle A4 centre (5.9309, -158.75) radius 2.161 projected
  circle A5 centre (5.9309, -6.35) radius 2.161 projected
  line L0 (0, 0) -> (11.1125, 0) projected
  line L1 (0, 0) -> (0, -215.9) projected
  line L2 (11.1125, -215.9) -> (0, -215.9) projected
  line L3 (11.1125, 0) -> (11.1125, -215.9) projected
  point P0 (17.1344, 0)
sketch "Sketch8" plane through (-7.4189, -0.1883, -209.55) normal (1, 0, 0) x (0, 0, -1)
  line L0 (-3.2283, 2.5775) -> (-3.2283, -2.5775)
  arc A0 (-3.2283, -2.5775) -> (-2.5775, -3.2283) centre (-2.5775, -2.5775) ccw
  arc A1 (-2.5775, 3.2283) -> (-3.2283, 2.5775) centre (-2.5775, 2.5775) ccw
  line L1 (2.5775, 3.2283) -> (-2.5775, 3.2283)
  arc A2 (3.2283, 2.5775) -> (2.5775, 3.2283) centre (2.5775, 2.5775) ccw
  line L2 (3.2283, -2.5775) -> (3.2283, 2.5775)
  arc A3 (2.5775, -3.2283) -> (3.2283, -2.5775) centre (2.5775, -2.5775) ccw
  line L3 (-2.5775, -3.2283) -> (2.5775, -3.2283)
  circle A4 centre (0, 0) radius 2.032
  circle A5 centre (0, 0) radius 5.08 projected
  point P0 (-209.55, 0.1883)
  constraints: 8 end point, 8 point on circle, 5 centre point
extrude "Extrusion6" cut sketch "Sketch8" against normal blind 3.81 contours A1 L1 A2 L2 A3 L3 A0 L0 | A4
sketch "Sketch9" plane through (-18.7219, -5.3699, 0) normal (-1, 0, 0) x (0, 0, 1)
  line L0 (-208.5975, 7.4041) -> (-210.5025, 7.4041) projected
  arc A0 (-210.5025, 7.4041) -> (-211.7725, 6.1341) centre (-210.5025, 6.1341) ccw projected
  line L1 (-211.7725, 6.1341) -> (-211.7725, 4.2291) projected
  arc A1 (-211.7725, 4.2291) -> (-210.5025, 2.9591) centre (-210.5025, 4.2291) ccw projected
  line L2 (-210.5025, 2.9591) -> (-208.5975, 2.9591) projected
  arc A2 (-208.5975, 2.9591) -> (-207.3275, 4.2291) centre (-208.5975, 4.2291) ccw projected
  line L3 (-207.3275, 4.2291) -> (-207.3275, 6.1341) projected
  arc A3 (-207.3275, 6.1341) -> (-208.5975, 7.4041) centre (-208.5975, 6.1341) ccw projected
  point P0 (0, 5.3699)
extrude "Extrusion7" cut sketch "Sketch9" against normal up to surface (1.5875 mm away)
sketch "Sketch10" plane through (-11.2289, -0.1883, -209.55) normal (1, 0, 0) x (0, 0, -1)
  arc A0 (-3.2283, -2.5775) -> (-2.5775, -3.2283) centre (-2.5775, -2.5775) ccw projected
  line L0 (2.5775, -3.2283) -> (-2.5775, -3.2283) projected
  arc A1 (2.5775, -3.2283) -> (3.2283, -2.5775) centre (2.5775, -2.5775) ccw projected
  line L1 (3.2283, 2.5775) -> (3.2283, -2.5775) projected
  arc A2 (3.2283, 2.5775) -> (2.5775, 3.2283) centre (2.5775, 2.5775) ccw projected
  line L2 (-2.5775, 3.2283) -> (2.5775, 3.2283) projected
  arc A3 (-2.5775, 3.2283) -> (-3.2283, 2.5775) centre (-2.5775, 2.5775) ccw projected
  line L3 (-3.2283, -2.5775) -> (-3.2283, 2.5775) projected
  circle A4 centre (0, 0) radius 2.0955
  point P0 (-209.55, 0.1883)
  dimension "d41" = 4.191
  constraints: 1 centre point
  measures "d41" diameter of A4
extrude "Extrusion8" cut sketch "Sketch10" along normal through all both and the other way through all contours A4
body "Solid1"
